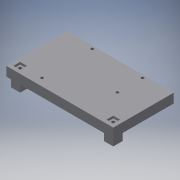
# Autodesk Inventor part: base_plate
Saved by Autodesk Inventor 2018 (Build 220112000, 112)
## iProperties
Created: 2020-02-21
Part Number: base_plate
Material: Generic
Document SubType Name: Modeling
Designer: bitbots
Density: 1 g/cm^3
Appearance: Default
Author: bitbots
Autodesk Inventor part; units mm, degrees
ref_plane "YZ Plane" through (0, 0, 0) normal (1, 0, 0) x (0, 1, 0)
ref_plane "XZ Plane" through (0, 0, 0) normal (0, 1, 0) x (-1, 0, 0)
ref_plane "XY Plane" through (0, 0, 0) normal (0, 0, 1) x (1, 0, 0)
sketch "Sketch1" plane through (0, 0, 0) normal (0, 0, 1) x (1, 0, 0)
  circle A0 centre (0, 13.5) radius 2 projected
  circle A1 centre (-100, 13.5) radius 2 projected
  line L0 (-100, 13.5) -> (-105, 13.5) construction
  line L1 (-100, 13.5) -> (-95, 13.5) construction
  line L2 (-105, 13.5) -> (-105, 8.5) construction
  line L3 (-105, 8.5) -> (-95, 8.5)
  line L4 (-95, 8.5) -> (-95, 18.5)
  line L5 (-95, 18.5) -> (-105, 18.5)
  line L6 (-105, 18.5) -> (-105, 8.5)
  line L7 (-5, 8.5) -> (5, 8.5)
  line L8 (5, 8.5) -> (5, 18.5)
  line L9 (5, 18.5) -> (-5, 18.5)
  line L10 (-5, 18.5) -> (-5, 8.5)
  line L11 (-5, 8.5) -> (5, 18.5) construction
  line L12 (5, 8.5) -> (-5, 18.5) construction
  point P0 (0, 0)
  dimension "d0" = 5
  dimension "d1" = 180
  dimension "d2" = 5
  dimension "d3" = 90
  dimension "d4" = 10
  dimension "d5" = 10
  dimension "d6" = 10
  dimension "d7" = 10
  constraints: 26 end point, 4 horizontal, 4 parallel, 3 perpendicular, 2 midpoint, 1 collinear
  measures "d0" distance of L0.start L0.end
  measures "d1" angle of L0 L1
  measures "d2" distance of L0.end L2.end
  measures "d3" angle of L2 L0
  measures "d4" distance of L5.end L4.end
  measures "d5" distance of L4.end L3.end
  measures "d6" distance of L9.end L8.end
  measures "d7" distance of L8.end L7.end
extrude "Extrusion1" add sketch "Sketch1" along normal blind 10
sketch "Sketch2" plane through (0, 0, 10) normal (0, 0, 1) x (1, 0, 0)
  circle A0 centre (-100, 13.5) radius 2 projected
  line L0 (-105, 8.5) -> (-95, 8.5) projected
  line L1 (-95, 8.5) -> (-95, 18.5) projected
  line L2 (-95, 18.5) -> (-105, 18.5) construction
  line L3 (-105, 18.5) -> (-105, 8.5) projected
  line L4 (-92.5, 21) -> (-107.5, 21) construction
  line L5 (-107.5, 21) -> (-107.5, 6) construction
  line L6 (-107.5, 6) -> (-92.5, 6) construction
  line L7 (-92.5, 6) -> (-92.5, 21) construction
  circle A1 centre (-100, 13.5) radius 2 construction
  line L8 (-92.5, 21) -> (-107.5, 6) construction
  line L9 (-107.5, 21) -> (-92.5, 6) construction
  line L10 (-107.5, 6) -> (7.5, 6)
  line L11 (7.5, 6) -> (7.5, 71)
  line L12 (7.5, 71) -> (-107.5, 71)
  line L13 (-107.5, 71) -> (-107.5, 6)
  circle A2 centre (0, 13.5) radius 2 projected
  point P0 (0, 0)
  dimension "d10" = 15
  dimension "d11" = 15
  dimension "d12" = 115
  dimension "d13" = 65
  constraints: 20 end point, 4 parallel, 2 horizontal, 2 midpoint, 2 perpendicular
  measures "d10" distance of L6.end L5.end
  measures "d11" distance of L5.end L4.end
  measures "d12" distance of L12.end L11.end
  measures "d13" distance of L11.end L10.end
extrude "Extrusion2" add sketch "Sketch2" along normal blind 10
sketch "Sketch3" plane through (0, 0, 20) normal (0, 0, 1) x (1, 0, 0)
  circle A0 centre (-100, 13.5) radius 2 construction
  circle A1 centre (0, 13.5) radius 2 construction
  line L0 (-103.6, 17.1) -> (-96.4, 17.1)
  line L1 (-96.4, 17.1) -> (-96.4, 9.9)
  line L2 (-96.4, 9.9) -> (-103.6, 9.9)
  line L3 (-103.6, 9.9) -> (-103.6, 17.1)
  line L4 (-103.6, 17.1) -> (-96.4, 9.9) construction
  line L5 (-96.4, 17.1) -> (-103.6, 9.9) construction
  line L6 (-3.6, 17.1) -> (3.6, 17.1)
  line L7 (3.6, 17.1) -> (3.6, 9.9)
  line L8 (3.6, 9.9) -> (-3.6, 9.9)
  line L9 (-3.6, 9.9) -> (-3.6, 17.1)
  line L10 (-3.6, 17.1) -> (3.6, 9.9) construction
  line L11 (3.6, 17.1) -> (-3.6, 9.9) construction
  point P0 (0, 0)
  dimension "d16" = 7.2
  dimension "d17" = 7.2
  dimension "d18" = 7.2
  dimension "d19" = 7.2
  constraints: 24 end point, 4 midpoint, 4 parallel, 2 horizontal, 2 perpendicular
  measures "d16" distance of L1.end L2.end
  measures "d17" distance of L0.end L1.end
  measures "d18" distance of L7.end L8.end
  measures "d19" distance of L6.end L7.end
extrude "Extrusion3" cut sketch "Sketch3" against normal blind 2.5
sketch "Sketch4" plane through (0, 0, 10) normal (0, 0, -1) x (-1, 0, 0)
  line L0 (-7.5, 6) -> (-7.5, 71) construction
  line L1 (-7.5, 71) -> (20, 71) construction
  line L2 (-7.5, 71) -> (107.5, 71) construction
  line L3 (20, 71) -> (23, 71) construction
  line L4 (23, 71) -> (23, 68) construction
  line L5 (23, 68) -> (20, 68) construction
  line L6 (20, 68) -> (20, 71) construction
  line L7 (23, 68) -> (77, 68) construction
  line L8 (77, 68) -> (77, 14) construction
  line L9 (23, 68) -> (23, 41) construction
  line L10 (23, 68) -> (50, 68) construction
  circle A0 centre (77, 68) radius 1.5
  circle A1 centre (77, 14) radius 1.5
  circle A2 centre (23, 68) radius 1.5
  circle A3 centre (23, 41) radius 1.5
  point P0 (0, 0)
  dimension "d22" = 27.5
  dimension "d23" = 3
  dimension "d24" = 3
  dimension "d25" = 54
  dimension "d26" = 54
  dimension "d27" = 90
  dimension "d28" = 27
  dimension "d29" = 90
  dimension "d30" = 3
  dimension "d31" = 3
  dimension "d32" = 3
  dimension "d33" = 3
  constraints: 18 end point, 4 centre point, 4 coincident, 3 parallel, 3 perpendicular, 2 horizontal, 1 point on line, 1 vertical
  measures "d22" distance of L0.end L1.end
  measures "d23" distance of L4.end L5.end
  measures "d24" distance of L3.end L4.end
  measures "d25" distance of L4.end L7.end
  measures "d26" distance of L7.end L8.end
  measures "d27" angle of L7 L8
  measures "d28" distance of L4.end L9.end
  measures "d29" angle of L9 L10
  measures "d30" diameter of A0
  measures "d31" diameter of A1
  measures "d32" diameter of A2
  measures "d33" diameter of A3
extrude "Extrusion4" cut sketch "Sketch4" against normal up to surface (10 mm away)
body "Solid1"
